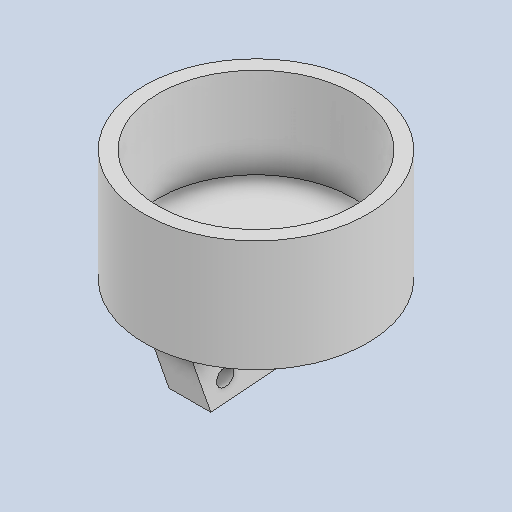
# Autodesk Inventor part: fixer
Saved by Autodesk Inventor 2025 (Build 290162000, 162)
## iProperties
Created: 2025-08-06
Part Number: fixer
Material: Generic
Document SubType Name: Modeling
Designer: Pravoslav
Density: 1 g/cm^3
Appearance: Default
Author: Pravoslav
Autodesk Inventor part; units mm, degrees
ref_plane "XZ Plane" through (0, 0, 0) normal (0, 1, 0) x (-1, 0, 0)
ref_plane "XY Plane" through (0, 0, 0) normal (0, 0, 1) x (1, 0, 0)
sketch "Sketch1" plane through (0, 0, 0) normal (0, 1, 0) x (-1, 0, 0)
  circle A0 centre (0, 0) radius 14
  circle A1 centre (0, 0) radius 16
  dimension "d0" = 28
  dimension "d1" = 32
  constraints: 2 centre point, 2 coincident
  measures "d0" diameter of A0
  measures "d1" diameter of A1
extrude "Extrusion1" add sketch "Sketch1" along normal blind 13
extrude "Extrusion2" add sketch "Sketch1" against normal blind 3 contours A0 | A1
ref_plane "Work Plane2" through (0, 0, 0) normal (1, 0, 0) x (0, 1, 0)
ref_plane "Work Plane1" through (16, 0, 0) normal (1, 0, 0) x (0, 1, 0)
sketch "Sketch3" plane through (0, 0, 0) normal (1, 0, 0) x (0, 1, 0)
  line L0 (-3, 16) -> (-3, -16) projected
  line L1 (-3, 0) -> (-10, 0)
  line L2 (-3, 0) -> (-39.281, 0)
  circle A0 centre (-39.281, 0) radius 34
  circle A1 centre (-39.281, 0) radius 31.5
  circle A2 centre (-39.281, 0) radius 29
  circle A3 centre (-8.9967, 0) radius 1.25
  circle A4 centre (-9.9967, 7.4154) radius 1.25
  line L3 (-3, -3.9193) -> (-12.3535, -3.7293)
  line L4 (-12.3535, -3.7293) -> (-13.3667, 9.4734)
  line L5 (-13.3667, 9.4734) -> (-3, 13.0827)
  point P0 (0, 0)
  dimension "d16" = 7
  dimension "d17" = 36.281
  dimension "d18" = 68
  dimension "d19" = 63
  dimension "d20" = 58
  dimension "d21" = 2.5
  dimension "d22" = 2.5
  constraints: 10 end point, 5 centre point, 3 coincident, 3 point on line, 2 horizontal, 1 midpoint
  measures "d16" distance of L1.start L1.end
  measures "d17" distance of L1.start L2.end
  measures "d18" diameter of A0
  measures "d19" diameter of A1
  measures "d20" diameter of A2
  measures "d21" diameter of A3
  measures "d22" diameter of A4
extrude "Extrusion4" add sketch "Sketch3" along normal mid plane 6 contours L0 L1 A0 L5 | L0 L3 A0 L1 | A0 L1 A3 A1 L5 | A0 L3 A1 A3 L1 | A1 A3 L2 A2 A4 L5 | L3 A2 L2 A3 A1 | A2 A4 L2 L4 L5 | L3 L4 L2 A2
body "Solid1"
